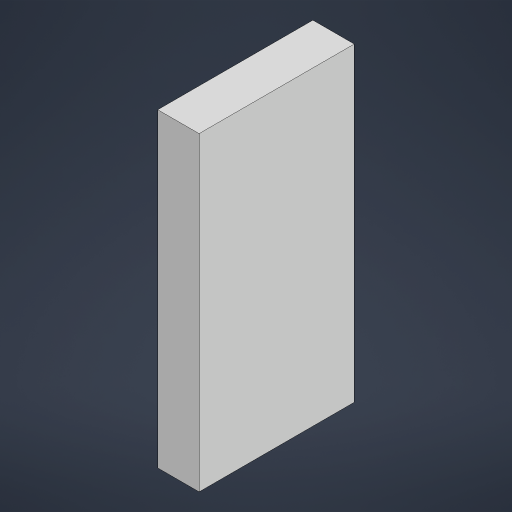
# Autodesk Inventor part: BallSensor_Mount
Saved by Autodesk Inventor 2024.2 (Build 282272000, 272)
## iProperties
Created: 2023-12-21
Part Number: BallSensor_Mount
Material: 一般
Document SubType Name: Modeling
Designer: Hanaoka
Density: 1 g/cm^3
Appearance: 既定
Author: Hanaoka
Autodesk Inventor part; units mm, degrees
ref_plane "YZ Plane" through (0, 0, 0) normal (1, 0, 0) x (0, 1, 0)
ref_plane "XZ Plane" through (0, 0, 0) normal (0, 1, 0) x (-1, 0, 0)
ref_plane "XY Plane" through (0, 0, 0) normal (0, 0, 1) x (1, 0, 0)
sketch "スケッチ1" plane through (0, 0, 0) normal (0, 1, 0) x (-1, 0, 0)
  line L0 (-2, 7.5) -> (2, 7.5)
  line L1 (2, 7.5) -> (2, -7.5)
  line L2 (2, -7.5) -> (-2, -7.5)
  line L3 (-2, -7.5) -> (-2, 7.5)
  line L4 (-2, 7.5) -> (2, -7.5) construction
  line L5 (2, 7.5) -> (-2, -7.5) construction
  circle A0 centre (0, 5.5) radius 1
  circle A1 centre (0, -5.5) radius 1
  line L6 (0, 5.5) -> (0, 7.5) construction
  line L7 (0, -5.5) -> (0, -7.5) construction
  point P0 (0, 0)
  dimension "d0" = 4
  dimension "d1" = 15
  dimension "d2" = 2
  dimension "d3" = 2
  constraints: 16 end point, 4 midpoint, 2 centre point, 2 parallel, 2 vertical, 1 collinear, 1 equal radius, 1 horizontal, 1 perpendicular
  measures "d0" distance of L1.end L2.end
  measures "d1" distance of L0.end L1.end
  measures "d2" diameter of A0
  measures "d3" distance of L6.start L6.end
extrude "押し出し1" add sketch "スケッチ1" along normal blind 30 contours L0 L1 L2 L3 | A0 | A1
extrude "押し出し2" cut sketch "スケッチ1" along normal blind 6 contours A0 | A1
